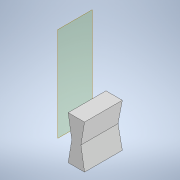
# Autodesk Inventor part: key
Saved by Autodesk Inventor 2022 (Build 260153000, 153)
## iProperties
Created: 2021-09-22
Part Number: key
Material: Generic
Document SubType Name: Modeling
Designer: tecware
Density: 1 g/cm^3
Appearance: Default
Author: tecware
## iProperties of the stored document key_3DPrint.ipt
Created: 2021-09-22
Part Number: key_3DPrint
Material: Generic
Document SubType Name: Modeling
Designer: tecware
Density: 1 g/cm^3
Appearance: Default
Author: tecware
Autodesk Inventor part; units mm, degrees
ref_plane "YZ Plane" through (0, 0, 0) normal (1, 0, 0) x (0, 1, 0)
ref_plane "XZ Plane" through (0, 0, 0) normal (0, 1, 0) x (-1, 0, 0)
ref_plane "XY Plane" through (0, 0, 0) normal (0, 0, 1) x (1, 0, 0)
sketch "Sketch1" plane through (0, 0, 0) normal (0, 0, 1) x (1, 0, 0)
  line L0 (-8, -8) -> (-8.6667, -4) projected
  line L1 (-8.6667, -4) -> (-5.3333, -4) projected
  line L2 (-5.3333, -4) -> (-6, -8) projected
  line L3 (10, -8) -> (-10, -8) projected
  line L4 (-8, -8) -> (-8.6667, -12)
  line L5 (-8.6667, -12) -> (-5.3333, -12)
  line L6 (-5.3333, -12) -> (-6, -8)
  line L7 (-7, -8) -> (-7.0726, -4.2007)
  line L8 (-7, -8) -> (-7.8, -8)
  line L9 (-7, -8) -> (-6.2, -8)
  line L10 (-7.8, -8) -> (-8.4332, -4.2007)
  line L11 (-8.4332, -4.2007) -> (-7.0726, -4.2007)
  line L12 (-6.2, -8) -> (-5.5668, -4.2007)
  line L13 (-5.5668, -4.2007) -> (-7.0726, -4.2007)
  line L14 (-7, -8) -> (-7.0726, -11.7993)
  line L15 (-7.8, -8) -> (-8.4332, -11.7993)
  line L16 (-8.4332, -11.7993) -> (-7.0726, -11.7993)
  line L17 (-6.2, -8) -> (-5.5668, -11.7993)
  line L18 (-5.5668, -11.7993) -> (-7.0726, -11.7993)
  point P0 (0, 0)
  dimension "d2" = 3.8
  dimension "d3" = 0.8
  dimension "d4" = 0.8
  constraints: 30 end point, 5 symmetric about line, 3 point on line, 2 horizontal, 2 parallel
  measures "d2" distance of L7.start L7.end
  measures "d3" distance of L7.start L8.end
  measures "d4" distance of L7.start L9.end
ref_plane "Work Plane1" through (-10, -8, -5.5) normal (0, 0, -1) x (0, 1, 0)
extrude "Extrusion1" add sketch "Sketch1" against normal blind 7 contours L10 L11 L7 L3 | L3 L14 L16 L15 | L7 L13 L12 L3 | L3 L17 L18 L14
ref_plane "Work Plane2" through (-10, -8, 0) normal (-1, 0, 0) x (0, 1, 0)
sketch "Sketch2" plane through (-10, -8, 0) normal (-1, 0, 0) x (0, 1, 0)
  line L0 (3.7993, 0) -> (3.7993, 7) projected
  line L1 (0, 0) -> (0, 7) projected
  line L2 (-3.7993, 0) -> (-3.7993, 7) projected
  line L3 (15, 7) -> (0, 6.5) projected
  line L4 (0, 7) -> (3.7993, 7) projected
  line L5 (3.7993, 7) -> (0, 7)
  line L6 (-3.7993, 0) -> (-3.7993, 7)
  line L7 (-15, 7) -> (0, 6.5)
  line L8 (0, 7) -> (-3.7993, 7)
  point P0 (8, 0)
  point P1 (-3.7993, 6.6266)
  point P2 (3.7993, 6.6266)
  constraints: 8 end point, 1 collinear, 1 symmetric about line
extrude "Extrusion2" cut sketch "Sketch2" against normal through all
body "Solid1"
